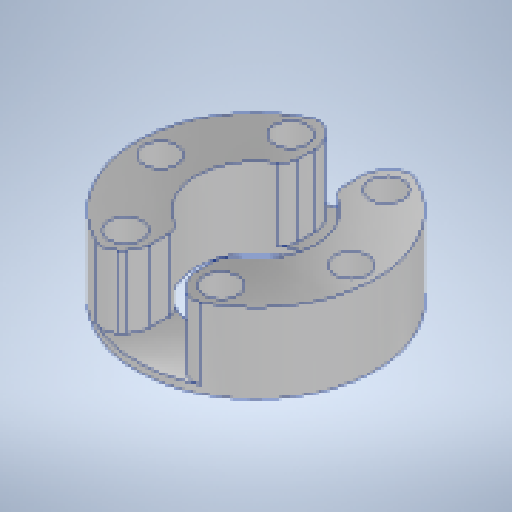
# Autodesk Inventor part: servoplate_forR2
Saved by Autodesk Inventor 2024 (Build 280153000, 153)
## iProperties
Created: 2025-05-24
Part Number: servoplate_forR2
Material: アルミニウム 6061
Document SubType Name: Modeling
Designer: kshau
Density: 2.7 g/cm^3
Appearance: アルミニウム - フラット
Author: kshau
Autodesk Inventor part; units mm, degrees
ref_plane "YZ Plane" through (0, 0, 0) normal (1, 0, 0) x (0, 1, 0)
ref_plane "XZ Plane" through (0, 0, 0) normal (0, 1, 0) x (-1, 0, 0)
ref_plane "XY Plane" through (0, 0, 0) normal (0, 0, 1) x (1, 0, 0)
sketch "スケッチ1" plane through (0, 0, 0) normal (0, 1, 0) x (-1, 0, 0)
  circle A0 centre (0, 0) radius 15
  dimension "d0" = 30
  constraints: 1 centre point, 1 coincident
  measures "d0" diameter of A0
extrude "押し出し1" add sketch "スケッチ1" along normal blind 10
sketch "スケッチ2" plane through (0, 10, 0) normal (0, 1, 0) x (1, 0, 0)
  circle A0 centre (0, 0) radius 12
  point P0 (-12, 0)
  point P1 (-6, -10.3923)
  point P2 (6, -10.3923)
  point P3 (12, 0)
  point P4 (6, 10.3923)
  point P5 (-6, 10.3923)
  dimension "d3" = 24
  dimension "d6" = 360
  constraints: 1 coincident, 1 horizontal alignment, 9 other
hole "穴1" at (-12, 10, 0) at (-6, 10, 10.3923) at (6, 10, 10.3923) at (12, 10, 0) at (6, 10, -10.3923) at (-6, 10, -10.3923) direction (0, -1, 0) diameter 4.2 end through all
sketch "スケッチ3" plane through (0, 10, 0) normal (0, 1, 0) x (1, 0, 0)
  circle A0 centre (0, 0) radius 7.5
  dimension "d15" = 15
  constraints: 1 centre point, 1 coincident
  measures "d15" diameter of A0
extrude "押し出し2" cut sketch "スケッチ3" against normal blind 10
sketch "スケッチ4" plane through (0, 10, 0) normal (0, 1, 0) x (1, 0, 0)
  circle A0 centre (-6, -10.3923) radius 2.1 projected
  circle A1 centre (6, -10.3923) radius 2.1 projected
  line L0 (-6, -10.3923) -> (6, -10.3923)
  circle A2 centre (-6, -10.3923) radius 3.1
  circle A3 centre (6, -10.3923) radius 3.1
  line L1 (-2.9, -10.3923) -> (-2.9, -6.9166)
  circle A4 centre (0, 0) radius 7.5 projected
  line L2 (2.9, -10.3923) -> (2.9, -6.9166)
  line L3 (-3.808, -12.5843) -> (-5.2681, -14.0445)
  circle A5 centre (0, 0) radius 15 projected
  line L4 (3.808, -12.5843) -> (5.2681, -14.0445)
  line L5 (-15, 0) -> (0, 0)
  circle A6 centre (-6, 10.3923) radius 3.1
  circle A7 centre (6, 10.3923) radius 3.1
  line L6 (-2.9, 10.3923) -> (-2.9, 6.9166)
  line L7 (2.9, 10.3923) -> (2.9, 6.9166)
  line L8 (-3.808, 12.5843) -> (-5.2681, 14.0445)
  line L9 (3.808, 12.5843) -> (5.2681, 14.0445)
  circle A8 centre (0, 0) radius 7.5
  circle A9 centre (0, 0) radius 15
  point P0 (-5.2681, 14.0445)
  dimension "d18" = 1
  dimension "d19" = 1
  dimension "d20" = 135
  constraints: 20 end point, 13 point on circle, 10 symmetric about line, 4 centre point, 4 coincident, 3 tangent, 2 horizontal, 2 point on line, 1 parallel, 1 perpendicular, 1 vertical, 8 other
  measures "d18" radial gap between concentric circles of A0 A2
  measures "d19" radial gap between concentric circles of A1 A3
  measures "d20" angle of L2 L4
extrude "押し出し3" cut sketch "スケッチ4" against normal blind 9 contours L1 A4 L2 L0 | L0 A3 L4 A5 L3 A2 | L6 A6 L8 A5 L9 A7 L7 A4
fillet "フィレット1" radius 2 8 edges at (5.2681, 5.5, -14.0445) (-5.2681, 5.5, -14.0445) (5.2681, 5.5, 14.0445) (-5.2681, 5.5, 14.0445) (-2.9, 5.5, -6.9166) (-2.9, 5.5, 6.9166) (2.9, 5.5, 6.9166) (2.9, 5.5, -6.9166)
sketch "スケッチ5" plane through (0, 1, 0) normal (0, 1, 0) x (1, 0, 0)
  arc A0 (-6.6047, -13.4677) -> (6.6047, -13.4677) centre (0, 0) ccw projected
  line L0 (-2.9, -10.3923) -> (-2.9, -8.1388) projected
  arc A1 (6.6047, -13.4677) -> (-6.6047, -13.4677) centre (0, 0) ccw projected
  circle A2 centre (0, 0) radius 15 projected
  line L1 (-6.1706, -13.672) -> (6.1706, -13.672)
  arc A3 (4.3098, -13.0862) -> (6.6047, -13.4677) centre (5.724, -11.672) ccw projected
  line L2 (6.1706, -13.672) -> (-6.1706, -13.672)
  line L3 (-6.1706, -13.672) -> (-6.1706, -24.6433)
  line L4 (-6.1706, -24.6433) -> (6.1706, -24.6433)
  line L5 (6.1706, -24.6433) -> (6.1706, -13.672)
  line L6 (-6.1706, -24.6433) -> (-15.2853, -20.5296)
  line L7 (-15.2853, -20.5296) -> (-10.7439, -10.4675)
  line L8 (-6.1706, -13.672) -> (-11.1715, -11.4149)
  point P0 (-10.7439, -10.4675)
  dimension "d28" = 10
  dimension "d29" = 10
  constraints: 16 end point, 3 parallel, 3 point on circle, 2 horizontal, 2 perpendicular, 2 point on line, 2 tangent
  measures "d28" distance between parallel lines of L8 L6
  measures "d29" distance of L3.end L6.end
extrude "押し出し4" [suppressed]
sketch "スケッチ6" plane through (0, 1, 0) normal (0, 1, 0) x (1, 0, 0)
  line L0 (-15.6324, -20.1472) -> (-7.4753, -3.7413) projected
  line L1 (-14.742, -18.3563) -> (-2.1859, -24.5993)
  line L2 (6.6781, -24.5993) -> (-6.6781, -24.5993) projected
  line L3 (-6.6781, -24.5993) -> (-15.6324, -20.1472) projected
  line L4 (-10.7006, -22.5993) -> (6.6781, -22.5993)
  line L5 (6.6781, 0) -> (6.6781, -24.5993) projected
  line L6 (-15.6324, -20.1472) -> (-6.6781, -24.5993) projected
  line L7 (-6.6781, -24.5993) -> (6.6781, -24.5993) projected
  line L8 (0, -24.5993) -> (0, -22.5993)
  point P0 (0, 0)
  point P1 (-15, 0)
  point P2 (-15, 0)
  point P3 (-6.2084, -22.5993)
  dimension "d33" = 2
  dimension "d34" = 2
  constraints: 6 end point, 3 point on line, 1 horizontal, 1 midpoint, 1 parallel, 1 perpendicular, 4 other
  measures "d33" distance between parallel lines of L7 L4
  measures "d34" distance between parallel lines of L6 L1
extrude "押し出し5" [suppressed]
